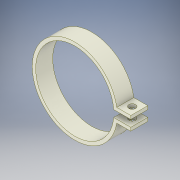
# Autodesk Inventor part: SupportBracket_BilgePumpMotor
Saved by Autodesk Inventor 2019 (Build 230136000, 136)
## iProperties
Created: 2019-03-02
Part Number: SupportBracket_BilgePumpMotor
Material: ABS Plastic
Document SubType Name: Modeling
Designer: User
Density: 1.06 g/cm^3
Appearance: Smooth - Ivory
Author: User
Autodesk Inventor part; units mm, degrees
ref_plane "YZ Plane" through (0, 0, 0) normal (1, 0, 0) x (0, 1, 0)
ref_plane "XZ Plane" through (0, 0, 0) normal (0, 1, 0) x (-1, 0, 0)
ref_plane "XY Plane" through (0, 0, 0) normal (0, 0, 1) x (1, 0, 0)
sketch "Sketch1" plane through (0, 0, 0) normal (0, 0, 1) x (1, 0, 0)
  arc A0 (22.9129, 2) -> (22.9129, -2) centre (0, 0) ccw
  arc A1 (24.6779, 4) -> (24.6779, -4) centre (0, 0) ccw
  line L0 (22.9129, 2) -> (24.9199, 2)
  line L1 (22.9129, -2) -> (24.9199, -2)
  line L2 (24.9199, 2) -> (32.9199, 2)
  line L3 (32.9199, 2) -> (32.9199, 4)
  line L4 (32.9199, 4) -> (24.6779, 4)
  line L5 (24.9199, -2) -> (32.9199, -2)
  line L6 (32.9199, -2) -> (32.9199, -4)
  line L7 (32.9199, -4) -> (24.6779, -4)
  dimension "d0" = 46
  dimension "d1" = 50
  dimension "d7" = 2
  dimension "d9" = 2
  constraints: 16 end point, 4 point on circle, 2 centre point, 2 coincident, 2 horizontal, 2 parallel, 2 perpendicular
  measures "d0" diameter of A0
  measures "d1" diameter of A1
  measures "d7" distance of L3.end L2.end
  measures "d9" distance of L5.end L6.end
extrude "Extrusion1" add sketch "Sketch1" against normal blind 10
sketch "Sketch2" plane through (24.6779, 4, 0) normal (0, 1, 0) x (1, 0, 0)
  line L0 (8.2419, 0) -> (0, 0) projected
  line L1 (8.2419, 0) -> (8.2419, 10) projected
  line L2 (0, 10) -> (8.2419, 10) projected
  line L3 (0, 0) -> (0, 10) projected
  circle A0 centre (4.121, 5) radius 2
  point P0 (-24.6779, 0)
  dimension "d12" = 4
  constraints: 1 centre point
  measures "d12" diameter of A0
extrude "Extrusion2" cut sketch "Sketch2" against normal blind 8.5 contours A0
body "Solid1"
